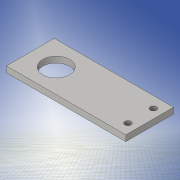
# Autodesk Inventor part: Pin Support Plate
Saved by Autodesk Inventor 2016 (Build 200138000, 138)
## iProperties
Created: 2015-08-05
Part Number: Pin Support Plate
Material: Generic
Document SubType Name: Modeling
Designer: Jason
Density: 1 g/cm^3
Appearance: Default
Author: Jason
Autodesk Inventor part; units mm, degrees
ref_plane "YZ Plane" through (0, 0, 0) normal (1, 0, 0) x (0, 1, 0)
ref_plane "XZ Plane" through (0, 0, 0) normal (0, 1, 0) x (-1, 0, 0)
ref_plane "XY Plane" through (0, 0, 0) normal (0, 0, 1) x (1, 0, 0)
sketch "Sketch1" plane through (0, 0, 0) normal (0, 1, 0) x (-1, 0, 0)
  line L0 (0, 0) -> (127, 0)
  line L1 (127, 0) -> (127, -50.8)
  line L2 (127, -50.8) -> (0, -50.8)
  line L3 (0, -50.8) -> (0, 0)
  dimension "d0" = 127
  dimension "d1" = 50.8
  constraints: 8 end point, 2 parallel, 1 horizontal, 1 perpendicular
  measures "d0" distance of L1.end L2.end
  measures "d1" distance of L2.end L0.start
extrude "Extrusion1" add sketch "Sketch1" along normal blind 6.35
sketch "Sketch2" plane through (0, 6.35, 0) normal (0, 1, 0) x (1, 0, 0)
  circle A0 centre (-99.441, 25.4) radius 14.2875
  line L0 (0, 0) -> (0, 50.8) projected
  dimension "d4" = 28.575
  dimension "d5" = 99.441
  constraints: 1 centre point
  measures "d4" diameter of A0
  measures "d5" distance from line of L0 A0.centre
extrude "Extrusion2" cut sketch "Sketch2" against normal blind 6.35
sketch "Sketch3" plane through (0, 6.35, 0) normal (0, 1, 0) x (1, 0, 0)
  line L0 (0, 0) -> (0, 50.8) projected
  line L1 (0, 0) -> (-9.525, 11.8364)
  line L2 (0, 50.8) -> (-9.525, 38.9636)
  dimension "d8" = 27.1272
  dimension "d9" = 9.525
  dimension "d10" = 9.525
  constraints: 4 end point, 1 equal length
  measures "d8" distance of L1.end L2.end
  measures "d9" distance from line of L0 L1.end
  measures "d10" distance from line of L0 L2.end
hole "Hole1" at (-9.525, 6.35, -11.8364) at (-9.525, 6.35, -38.9636) direction (0, -1, 0) diameter 6.5278 depth 25.4 tip angle 118
body "Solid1"
